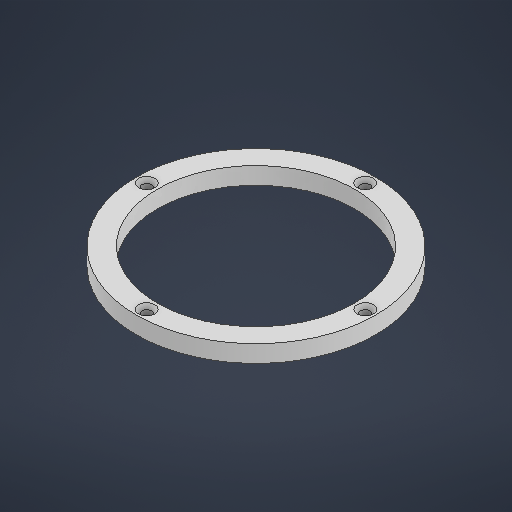
# Autodesk Inventor part: outerbearingwheel
Saved by Autodesk Inventor 2026 (Build 300175000, 175)
## iProperties
Created: 2026-04-15
Part Number: outerbearingwheel
Material: Generic
Document SubType Name: Modeling
Designer: CAD237 PC35
Density: 1 g/cm^3
Appearance: Default
Author: CAD237 PC35
Autodesk Inventor part; units mm, degrees
ref_plane "YZ Plane" through (0, 0, 0) normal (1, 0, 0) x (0, 1, 0)
ref_plane "XZ Plane" through (0, 0, 0) normal (0, 1, 0) x (-1, 0, 0)
ref_plane "XY Plane" through (0, 0, 0) normal (0, 0, 1) x (1, 0, 0)
sketch "Sketch1" plane through (0, 0, 0) normal (0, 1, 0) x (-1, 0, 0)
  circle A0 centre (0, 0) radius 70
  circle A1 centre (0, 0) radius 57.785
  dimension "d0" = 140
  dimension "d3" = 115.57
  constraints: 2 centre point, 1 coincident
  measures "d0" diameter of A0
  measures "d3" diameter of A1
extrude "Extrusion1" add sketch "Sketch1" along normal blind 10
sketch "Sketch2" plane through (0, 10, 0) normal (0, 1, 0) x (1, 0, 0)
  circle A0 centre (0, 0) radius 70 projected
  circle A1 centre (0, 0) radius 57.785 projected
  circle A2 centre (0, 0) radius 70 projected
  line L0 (0, 0) -> (-64.008, 0)
  line L1 (0, 0) -> (0, -64.008)
  point P0 (0, -64.008)
  point P1 (64.008, 0)
  point P2 (0, 64.008)
  dimension "d24" = 64.008
  dimension "d25" = 64.008
  dimension "d28" = 360
  constraints: 4 end point, 2 coincident, 1 horizontal, 1 perpendicular, 5 other
  measures "d24" distance of L0.start L0.end
  measures "d25" distance of L0.start L1.end
hole "Hole2" at (-64.008, 10, 0) at (0, 10, -64.008) at (64.008, 10, 0) at (0, 10, 64.008) direction (0, -1, 0) diameter 5.7 end through all countersink diameter 9.525 countersink angle 82
body "Solid1"
